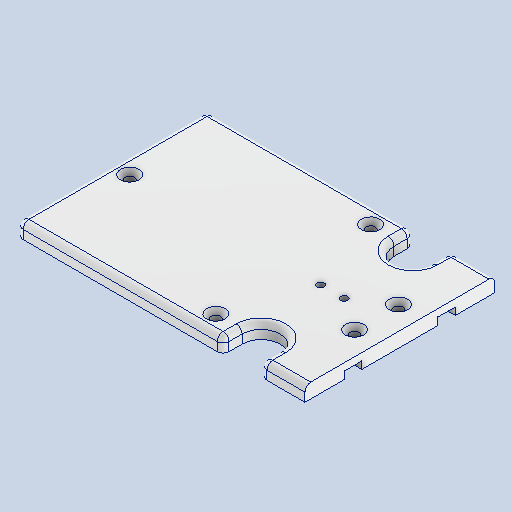
# Autodesk Inventor part: SchlittenDeckel
Saved by Autodesk Inventor 2025 (Build 290162010, 162A)
## iProperties
Created: 2024-11-26
Part Number: SchlittenDeckel
Material: Aluminium 6061(1)
Document SubType Name: Modeling
Designer: Admin
Density: 2.7 g/cm^3
Appearance: Aluminium - flach(1)
Author: Admin
Autodesk Inventor part; units mm, degrees
ref_plane "YZ Plane" through (0, 0, 0) normal (1, 0, 0) x (0, 1, 0)
ref_plane "XZ Plane" through (0, 0, 0) normal (0, 1, 0) x (-1, 0, 0)
ref_plane "XY Plane" through (0, 0, 0) normal (0, 0, 1) x (1, 0, 0)
sketch "Skizze1" plane through (0, 0, 0) normal (0, 0, 1) x (1, 0, 0)
  line L0 (0, -65) -> (98.5, -65)
  line L1 (0, 0) -> (0, -65)
  line L2 (98.5, 0) -> (0, 0)
  line L3 (98.5, -65) -> (98.5, 0)
  line L4 (70.5, -58.5) -> (70.5, -65)
  line L5 (83.5, -58.5) -> (83.5, -65)
  line L6 (0, -65) -> (77, -65)
  arc A0 (77, 0) -> (77, -13) centre (77, -6.5) ccw
  arc A1 (77, -52) -> (77, -65) centre (77, -58.5) ccw
  arc A2 (77, -65) -> (77, -52) centre (77, -58.5) ccw
  arc A3 (77, -13) -> (77, 0) centre (77, -6.5) ccw
  line L7 (83.5, -6.5) -> (83.5, 0)
  line L8 (70.5, -6.5) -> (70.5, 0)
  arc A4 (77, 0) -> (77, -13) centre (77, -6.5) ccw
  arc A5 (77, -13) -> (77, 0) centre (77, -6.5) ccw
  line L9 (2, -65) -> (77, -65)
  arc A6 (77, -52) -> (77, -65) centre (77, -58.5) ccw
  arc A7 (77, -65) -> (77, -52) centre (77, -58.5) ccw
  point P0 (78.5905, -65)
  point P1 (82, -65)
  point P2 (83.5, -58.5)
  dimension "d87" = 15
  constraints: 25 point on circle, 20 end point, 8 centre point, 7 perpendicular, 5 point on line, 3 coincident, 2 horizontal, 2 tangent, 12 other
  measures "d87" distance from line of point (83.5, -58.5) L3
extrude "Extrusion1" add sketch "Skizze1" along normal blind 5 contours L1 L2 L8 A0 A3 L7 L3 L0 L5 A2 A1 L4
sketch "Skizze2" plane through (0, 0, 0) normal (0, 0, -1) x (-1, 0, 0)
  circle A0 centre (-49, -13) radius 1 projected
  circle A1 centre (-35.6667, -52) radius 1 projected
  circle A2 centre (-22.3333, -49) radius 1 projected
  circle A3 centre (-9, -16) radius 1 projected
  point P0 (0, 0)
hole "umlenkpins" at (49, -13, 0) at (35.6667, -52, 0) at (22.3333, -49, 0) at (9, -16, 0) direction (0, 0, 1) diameter 2 depth 3 tip angle 118
sketch "Skizze8" plane through (98.5, -58.5, 0) normal (1, 0, 0) x (0, 0, -1)
  line L0 (0, -6.5) -> (0, 58.5) projected
  line L1 (0, 7) -> (-2.5, 7)
  line L2 (-2.5, 7) -> (-2.5, 13)
  line L3 (-2.5, 13) -> (0, 13)
  line L4 (0, 13) -> (0, 7)
  line L5 (0, 26) -> (-5, 26) construction
  line L6 (-5, -6.5) -> (-5, 58.5) construction
  line L7 (0, 45) -> (-2.5, 45)
  line L8 (-2.5, 45) -> (-2.5, 39)
  line L9 (-2.5, 39) -> (0, 39)
  line L10 (0, 39) -> (0, 45)
  point P0 (0, 0)
  point P1 (0, 52)
  point P2 (-5, 0)
  point P3 (-5, 52)
  point P4 (0, 39)
  point P5 (0, 45)
  point P6 (0, 13)
  dimension "d59" = 2.5
  dimension "d60" = 6
  dimension "d61" = 13
  constraints: 18 end point, 4 symmetric about line, 2 midpoint, 2 parallel, 1 horizontal, 1 perpendicular, 1 point on line
  measures "d59" distance of L2.end L3.end
  measures "d60" distance of L1.end L2.end
  measures "d61" distance between parallel lines of L5 L3
extrude "Extrusion4" cut sketch "Skizze8" against normal blind 3
fillet "Rundung2" radius 2 17 edges at (91, 0, 5) (35.25, 0, 5) (91, -65, 5) (35.25, -65, 5) (0, -32.5, 5) (0, 0, 2.5) (0, -65, 2.5) (70.5, -65, 2.5) (83.5, -65, 2.5) (77, -52, 5) (83.5, -61.75, 5) (70.5, -61.75, 5) (70.5, -3.25, 5) (83.5, -3.25, 5) (77, -13, 5) (70.5, 0, 2.5) (83.5, 0, 2.5)
sketch "Skizze9" plane through (0, 0, 5) normal (0, 0, 1) x (1, 0, 0)
  line L0 (2, -63) -> (2, -2) projected
  line L1 (2, -32.5) -> (6, -32.5)
  line L2 (2, -2) -> (68.5, -2) projected
  line L3 (62, -2) -> (62, -6)
  line L4 (62, -63) -> (62, -59)
  line L5 (68.5, -63) -> (2, -63) projected
  line L6 (90.5, -25) -> (90.5, -40)
  line L7 (90.5, -32.5) -> (98.5, -32.5)
  line L8 (98.5, -65) -> (98.5, 0) projected
  point P0 (0, 0)
  point P1 (138.5, -53.0228)
  point P2 (138.5, -11.9773)
  dimension "d65" = 4
  dimension "d66" = 60
  dimension "d67" = 15
  dimension "d88" = 8
  constraints: 10 end point, 3 coincident, 3 vertical, 2 horizontal, 2 midpoint, 2 perpendicular, 2 point on line, 1 collinear, 2 other
  measures "d65" distance of L1.start L1.end
  measures "d66" distance between parallel lines of L0 L3
  measures "d67" distance of L6.start L6.end
  measures "d88" distance of L7.start L7.end
hole "Bohrung5" at (6, -32.5, 5) at (62, -6, 5) at (62, -59, 5) at (90.5, -25, 5) at (90.5, -40, 5) direction (0, 0, -1) diameter 3.2 depth 7.8 tip angle 118 countersink diameter 6.3 countersink angle 90 clearance for "Flachkopfmaschinenschraube" size "M3" standard "ANSI Metrisches M Profil"
sketch "Skizze10" plane through (0, 0, 5) normal (0, 0, 1) x (1, 0, 0)
  circle A0 centre (65.05, -128.1464) radius 1.5696
  line L0 (65.05, -128.1464) -> (65.05, 71.8536) construction
  line L1 (31.95, -141.1464) -> (48.05, -141.1464) construction
  circle A1 centre (65.05, -32.5) radius 1 construction
  line L2 (2, -63) -> (2, -2) construction
  line L3 (2, -32.5) -> (65.05, -32.5) construction
  line L4 (65.05, -32.5) -> (71.434, -32.5) construction
  line L5 (71.434, -32.5) -> (79.434, -32.5) construction
  point P0 (0, 0)
  dimension "d75" = 90
  dimension "d76" = 2
  dimension "d77" = 8
  dimension "d78" = 6.384
  dimension "d79" = 200
  constraints: 10 end point, 2 centre point, 2 coincident, 2 horizontal, 2 point on line, 1 midpoint, 1 perpendicular, 1 vertical, 4 other
  measures "d75" angle of L0 L1
  measures "d76" diameter of A1
  measures "d77" distance of L4.end L5.end
  measures "d78" distance of L3.end L4.end
  measures "d79" distance of L0.start L0.end
hole "Bohrung6" at (79.434, -32.5, 5) at (71.434, -32.5, 5) direction (0, 0, -1) diameter 2.459 end through all thread size "M3x0.5" class "6H" standard "ANSI Metric M Profile"
